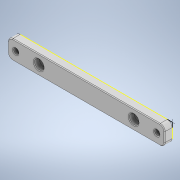
# Autodesk Inventor part: NEW_ACU_FIX1
Saved by Autodesk Inventor 2022 (Build 260153000, 153)
## iProperties
Created: 2021-11-12
Part Number: NEW_ACU_FIX1
Material: Generic
Document SubType Name: Modeling
Designer: Viktor
Density: 1 g/cm^3
Appearance: Default
Author: Viktor
Autodesk Inventor part; units mm, degrees
ref_plane "YZ Plane" through (0, 0, 0) normal (1, 0, 0) x (0, 1, 0)
ref_plane "XZ Plane" through (0, 0, 0) normal (0, 1, 0) x (-1, 0, 0)
ref_plane "XY Plane" through (0, 0, 0) normal (0, 0, 1) x (1, 0, 0)
sketch "Sketch1" plane through (0, 0, 0) normal (0, 0, 1) x (1, 0, 0)
  line L0 (-82.5, -10) -> (82.5, -10)
  line L1 (82.5, -10) -> (82.5, 10)
  line L2 (82.5, 10) -> (-82.5, 10)
  line L3 (-82.5, 10) -> (-82.5, -10)
  line L4 (-82.5, -10) -> (82.5, 10) construction
  line L5 (82.5, -10) -> (-82.5, 10) construction
  point P0 (0, 0)
  dimension "d0" = 165
  dimension "d1" = 20
  constraints: 12 end point, 2 midpoint, 2 parallel, 1 horizontal, 1 perpendicular
  measures "d0" distance of L1.end L2.end
  measures "d1" distance of L2.end L0.start
extrude "Extrusion1" add sketch "Sketch1" along normal blind 8
sketch "Sketch2" plane through (0, 0, 8) normal (0, 0, 1) x (1, 0, 0)
  line L0 (-115.5, 0) -> (115.5, 0) construction
  circle A0 centre (-50, 0) radius 5
  line L1 (0, 14) -> (0, -14) construction
  circle A1 centre (50, 0) radius 5
  point P0 (0, 0)
  dimension "d4" = 10
  dimension "d5" = 50
  constraints: 2 centre point, 1 point on line, 1 symmetric about line, 1 other
  measures "d4" diameter of A0
  measures "d5" distance from line of L1 A0.centre
extrude "Extrusion2" cut sketch "Sketch2" against normal blind 5.5
sketch "Sketch3" plane through (-50, 0, 2.5) normal (0, 0, 1) x (1, 0, 0)
  circle A0 centre (0, 0) radius 5 projected
  circle A1 centre (100, 0) radius 5 projected
  circle A2 centre (0, 0) radius 2.25
  circle A3 centre (100, 0) radius 2.25
  point P0 (50, 0)
  dimension "d8" = 4.5
  dimension "d9" = 4.5
  constraints: 2 centre point, 2 coincident
  measures "d8" diameter of A2
  measures "d9" diameter of A3
extrude "Extrusion3" cut sketch "Sketch3" against normal through all contours A2 | A3
sketch "Sketch4" plane through (0, 0, 0) normal (0, 0, -1) x (-1, 0, 0)
  line L0 (-115.5, 0) -> (115.5, 0) construction
  line L1 (0, -14) -> (0, 14) construction
  line L2 (78.5, -2.4249) -> (74.3, -4.8497)
  line L3 (74.3, -4.8497) -> (70.1, -2.4249)
  line L4 (70.1, -2.4249) -> (70.1, 2.4249)
  line L5 (70.1, 2.4249) -> (74.3, 4.8497)
  line L6 (74.3, 4.8497) -> (78.5, 2.4249)
  line L7 (78.5, 2.4249) -> (78.5, -2.4249)
  line L8 (82.5, 10) -> (82.5, -10) projected
  line L9 (-78.5, -2.4249) -> (-74.3, -4.8497)
  line L10 (-74.3, -4.8497) -> (-70.1, -2.4249)
  line L11 (-70.1, -2.4249) -> (-70.1, 2.4249)
  line L12 (-70.1, 2.4249) -> (-74.3, 4.8497)
  line L13 (-74.3, 4.8497) -> (-78.5, 2.4249)
  line L14 (-78.5, 2.4249) -> (-78.5, -2.4249)
  point P0 (0, 0)
  point P1 (74.3, 0)
  point P2 (-74.3, 0)
  dimension "d12" = 8.4
  dimension "d13" = 4
  constraints: 24 end point, 7 symmetric about line, 1 point on line, 1 vertical, 13 other
  measures "d12" distance between parallel lines of L7 L4
  measures "d13" distance between parallel lines of L8 L7
extrude "Extrusion4" cut sketch "Sketch4" against normal blind 3.8
sketch "Sketch5" plane through (0, 0, 3.8) normal (0, 0, -1) x (-1, 0, 0)
  line L0 (74.3, 4.8497) -> (78.5, 2.4249) projected
  line L1 (70.1, 2.4249) -> (74.3, 4.8497) projected
  line L2 (70.1, -2.4249) -> (70.1, 2.4249) projected
  line L3 (74.3, -4.8497) -> (70.1, -2.4249) projected
  line L4 (78.5, -2.4249) -> (74.3, -4.8497) projected
  line L5 (78.5, 2.4249) -> (78.5, -2.4249) projected
  line L6 (-70.1, -2.4249) -> (-74.3, -4.8497) projected
  line L7 (-70.1, 2.4249) -> (-70.1, -2.4249) projected
  line L8 (-74.3, 4.8497) -> (-70.1, 2.4249) projected
  line L9 (-78.5, 2.4249) -> (-74.3, 4.8497) projected
  line L10 (-78.5, -2.4249) -> (-78.5, 2.4249) projected
  line L11 (-74.3, -4.8497) -> (-78.5, -2.4249) projected
  line L12 (115.5, 0) -> (-115.5, 0) projected
  circle A0 centre (74.3, 0) radius 2.75
  line L13 (0, -14) -> (0, 14) projected
  line L14 (-74.3, 4.8497) -> (-78.5, 2.4249)
  line L15 (-70.1, 2.4249) -> (-74.3, 4.8497)
  line L16 (-70.1, -2.4249) -> (-70.1, 2.4249)
  line L17 (-74.3, -4.8497) -> (-70.1, -2.4249)
  line L18 (-78.5, -2.4249) -> (-74.3, -4.8497)
  line L19 (-78.5, 2.4249) -> (-78.5, -2.4249)
  circle A1 centre (-74.3, 0) radius 2.75
  point P0 (0, 0)
  dimension "d16" = 8.4
  dimension "d17" = 4.2
  dimension "d18" = 5.5
  constraints: 12 end point, 2 centre point, 1 point on line, 1 symmetric about line, 1 other
  measures "d16" distance between parallel lines of L2 L5
  measures "d17" distance from line of L5 A0.centre
  measures "d18" diameter of A0
extrude "Extrusion5" cut sketch "Sketch5" against normal through all contours A0 L12 | L12 A0 | A1 L12 | L12 A1
sketch "Sketch6" plane through (0, 0, 3.8) normal (0, 0, -1) x (-1, 0, 0)
  line L0 (74.3, -4.8497) -> (74.3, -10.0295) construction
  circle A0 centre (74.3, -3.5997) radius 1.25
  point P0 (0, 0)
  dimension "d21" = 2.5
  constraints: 2 end point, 1 point on line, 1 vertical, 1 vertical alignment, 2 other
extrude "Extrusion6" cut sketch "Sketch6" along normal up to surface (3.8 mm away)
pattern_circular "Circular Pattern1" count 6 over 360 about axis through (-74.3, 0, 3.8) along (0, 0, 1) of "Extrusion6"
mirror "Mirror1" about plane through (0, 0, 0) normal (1, 0, 0) of "Extrusion6", "Circular Pattern1"
fillet "Fillet1" radius 5 4 edges at (-82.5, 10, 4) (-82.5, -10, 4) (82.5, -10, 4) (82.5, 10, 4)
chamfer "Chamfer1" distance 0.75 angle 45 12 edges at (0, -10, 8) (81.0355, -8.5355, 8) (82.5, 0, 8) (81.0355, 8.5355, 8) (0, 10, 8) (-81.0355, 8.5355, 8) (-82.5, 0, 8) (-81.0355, -8.5355, 8) (-55, 0, 8) (45, 0, 8) (-71.55, 0, 8) (77.05, 0, 8)
sketch "Sketch7" plane through (0, 0, 0) normal (0, 0, -1) x (-1, 0, 0)
  line L0 (-77.5, 10) -> (77.5, 10) projected
  line L1 (-77.5, 10) -> (-82.5, 10)
  line L2 (-82.5, -5) -> (-82.5, 5) projected
  line L3 (-82.5, 10) -> (-82.5, 5)
  point P0 (0, 0)
  constraints: 4 end point, 1 coincident, 1 collinear, 1 horizontal
equation "\"d17\" = 0.5 * d16"
body "Solid1"
